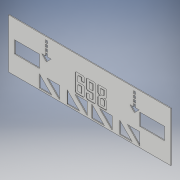
# Autodesk Inventor part: Lower Ramp
Saved by Autodesk Inventor 2018 (Build 220112000, 112)
## iProperties
Created: 2018-02-11
Part Number: Lower Ramp
Material: Generic
Document SubType Name: Modeling
Designer: Orangeracer
Density: 1 g/cm^3
Appearance: Default
Author: Orangeracer
Autodesk Inventor part; units mm, degrees
ref_plane "YZ Plane" through (0, 0, 0) normal (1, 0, 0) x (0, 1, 0)
ref_plane "XZ Plane" through (0, 0, 0) normal (0, 1, 0) x (-1, 0, 0)
ref_plane "XY Plane" through (0, 0, 0) normal (0, 0, 1) x (1, 0, 0)
sketch "Sketch1" plane through (0, 0, 0) normal (0, 0, 1) x (1, 0, 0)
  line L0 (0, 0) -> (666.75, 0)
  line L1 (666.75, 0) -> (666.75, -76.2)
  line L2 (666.75, -76.2) -> (0, -76.2)
  line L3 (0, -76.2) -> (0, 0)
  line L4 (127, 0) -> (539.75, 0)
  line L5 (539.75, 0) -> (539.75, 50.8)
  line L6 (539.75, 50.8) -> (127, 50.8)
  line L7 (127, 50.8) -> (127, 0)
  line L8 (0, 50.8) -> (666.75, 50.8)
  line L9 (666.75, 50.8) -> (666.75, 127)
  line L10 (666.75, 127) -> (0, 127)
  line L11 (0, 127) -> (0, 50.8)
  line L12 (25.4, 50.8) -> (0, 50.8)
  line L13 (0, 50.8) -> (0, 0)
  line L14 (0, 0) -> (25.4, 0)
  line L15 (25.4, 0) -> (25.4, 50.8)
  line L16 (666.75, 50.8) -> (641.35, 50.8)
  line L17 (641.35, 50.8) -> (641.35, 0)
  line L18 (641.35, 0) -> (666.75, 0)
  line L19 (666.75, 0) -> (666.75, 50.8)
  dimension "d0" = 666.75
  dimension "d1" = 76.2
  dimension "d2" = 50.8
  dimension "d3" = 666.75
  dimension "d4" = 0
  dimension "d5" = 76.2
  dimension "d6" = 127
  dimension "d7" = 127
  dimension "d8" = 25.4
  dimension "d9" = 50.8
  dimension "d10" = 25.4
  constraints: 40 end point, 10 parallel, 5 horizontal, 5 perpendicular, 4 point on line
  measures "d0" distance of L1.end L2.end
  measures "d1" distance of L0.end L1.end
  measures "d2" distance of L6.end L4.start
  measures "d3" distance of L9.end L10.end
  measures "d4" distance between parallel lines of L1 L9
  measures "d5" distance of L10.end L8.start
  measures "d6" distance between parallel lines of L3 L7
  measures "d7" distance between parallel lines of L9 L5
  measures "d8" distance between parallel lines of L13 L15
  measures "d9" distance of L12.end L0.start
  measures "d10" distance between parallel lines of L19 L17
extrude "Extrusion1" add sketch "Sketch1" along normal blind 3.175 contours L13 L8 L15 L0 | L0 L1 L2 L3 | L11 L10 L9 L8 L6 | L7 L6 L5 L0 | L0 L17 L8 L19
sketch "Sketch2" plane through (0, 0, 3.175) normal (0, 0, 1) x (1, 0, 0)
  line L0 (269.875, 63.5) -> (563.8865, 63.5) construction
  line L1 (563.8865, 63.5) -> (563.8865, -18.7489) construction
  line L2 (563.8865, -18.7489) -> (269.875, -18.7489) construction
  line L3 (269.875, -18.7489) -> (269.875, 63.5) construction
  line L4 (127, 50.8) -> (127, 0) projected
  line L5 (666.75, 127) -> (0, 127) projected
  spline S0 degree 2 poles (311.2942, -6.6857) (311.2942, -12.7) (305.2799, -12.7) knots 0 0 0 1 1 1
  line L6 (305.2799, -12.7) -> (280.4851, -12.7)
  spline S1 degree 2 poles (280.4851, -12.7) (274.4708, -12.7) (274.4708, -6.6857) knots 0 0 0 1 1 1
  line L7 (274.4708, -6.6857) -> (274.4708, 57.4857)
  spline S2 degree 2 poles (274.4708, 57.4857) (274.4708, 63.5) (280.3716, 63.5) knots 0 0 0 1 1 1
  line L8 (280.3716, 63.5) -> (305.053, 63.5)
  spline S3 degree 2 poles (305.053, 63.5) (311.124, 63.5) (311.124, 57.4857) knots 0 0 0 1 1 1
  line L9 (311.124, 57.4857) -> (311.124, 40.4074)
  line L10 (311.124, 40.4074) -> (299.9465, 40.4074)
  line L11 (299.9465, 40.4074) -> (299.9465, 53.741)
  line L12 (299.9465, 53.741) -> (285.6483, 53.741)
  line L13 (285.6483, 53.741) -> (285.6483, 30.8185)
  line L14 (285.6483, 30.8185) -> (305.2799, 30.8185)
  spline S4 degree 2 poles (305.2799, 30.8185) (311.2942, 30.8185) (311.2942, 24.8042) knots 0 0 0 1 1 1
  line L15 (311.2942, 24.8042) -> (311.2942, -6.6857)
  line L16 (300.1734, -2.941) -> (300.1734, 21.1162)
  line L17 (300.1734, 21.1162) -> (285.6483, 21.1162)
  line L18 (285.6483, 21.1162) -> (285.6483, -2.941)
  line L19 (285.6483, -2.941) -> (300.1734, -2.941)
  spline S5 degree 2 poles (357.139, -6.6857) (357.139, -12.7) (351.1247, -12.7) knots 0 0 0 1 1 1
  line L20 (351.1247, -12.7) -> (326.2165, -12.7)
  spline S6 degree 2 poles (326.2165, -12.7) (320.4859, -12.7) (320.4859, -6.6857) knots 0 0 0 1 1 1
  line L21 (320.4859, -6.6857) -> (320.4859, 10.3926)
  line L22 (320.4859, 10.3926) -> (331.6634, 10.3926)
  line L23 (331.6634, 10.3926) -> (331.6634, -2.941)
  line L24 (331.6634, -2.941) -> (345.848, -2.941)
  line L25 (345.848, -2.941) -> (345.848, 19.9815)
  line L26 (345.848, 19.9815) -> (325.8193, 19.9815)
  spline S7 degree 2 poles (325.8193, 19.9815) (320.2022, 19.9815) (320.2022, 25.9958) knots 0 0 0 1 1 1
  line L27 (320.2022, 25.9958) -> (320.2022, 57.4857)
  spline S8 degree 2 poles (320.2022, 57.4857) (320.2022, 63.5) (325.8193, 63.5) knots 0 0 0 1 1 1
  line L28 (325.8193, 63.5) -> (351.0113, 63.5)
  spline S9 degree 2 poles (351.0113, 63.5) (357.139, 63.5) (357.139, 57.4857) knots 0 0 0 1 1 1
  line L29 (357.139, 57.4857) -> (357.139, -6.6857)
  line L30 (345.848, 29.627) -> (345.848, 53.741)
  line L31 (345.848, 53.741) -> (331.323, 53.741)
  line L32 (331.323, 53.741) -> (331.323, 29.627)
  line L33 (331.323, 29.627) -> (345.848, 29.627)
  spline S10 degree 2 poles (403.9484, -6.6857) (403.9484, -12.7) (397.9341, -12.7) knots 0 0 0 1 1 1
  line L34 (397.9341, -12.7) -> (372.2883, -12.7)
  spline S11 degree 2 poles (372.2883, -12.7) (366.274, -12.7) (366.274, -6.6857) knots 0 0 0 1 1 1
  line L35 (366.274, -6.6857) -> (366.274, 16.4069)
  spline S12 degree 2 poles (366.274, 16.4069) (366.274, 20.6056) (369.1109, 22.8751) knots 0 0 0 1 1 1
  spline S13 degree 2 poles (369.1109, 22.8751) (372.4585, 24.8042) (375.8628, 26.7901) knots 0 0 0 1 1 1
  spline S14 degree 2 poles (375.8628, 26.7901) (372.5719, 28.6625) (369.3378, 30.5916) knots 0 0 0 1 1 1
  spline S15 degree 2 poles (369.3378, 30.5916) (366.3874, 32.9179) (366.3874, 36.8896) knots 0 0 0 1 1 1
  line L36 (366.3874, 36.8896) -> (366.3874, 57.4857)
  spline S16 degree 2 poles (366.3874, 57.4857) (366.3874, 63.5) (372.5719, 63.5) knots 0 0 0 1 1 1
  line L37 (372.5719, 63.5) -> (397.8206, 63.5)
  spline S17 degree 2 poles (397.8206, 63.5) (403.7782, 63.5) (403.7782, 57.4857) knots 0 0 0 1 1 1
  line L38 (403.7782, 57.4857) -> (403.7782, 36.8896)
  spline S18 degree 2 poles (403.7782, 36.8896) (403.7782, 32.8611) (400.8278, 30.5916) knots 0 0 0 1 1 1
  spline S19 degree 2 poles (400.8278, 30.5916) (397.5937, 28.6625) (394.3028, 26.7901) knots 0 0 0 1 1 1
  spline S20 degree 2 poles (394.3028, 26.7901) (397.6504, 24.8042) (401.0547, 22.8751) knots 0 0 0 1 1 1
  spline S21 degree 2 poles (401.0547, 22.8751) (403.9484, 20.6056) (403.9484, 16.4069) knots 0 0 0 1 1 1
  line L39 (403.9484, 16.4069) -> (403.9484, -6.6857)
  line L40 (392.6007, -3.1112) -> (392.6007, 17.9956)
  line L41 (392.6007, 17.9956) -> (385.1112, 22.3077)
  line L42 (385.1112, 22.3077) -> (377.5649, 17.9956)
  line L43 (377.5649, 17.9956) -> (377.5649, -3.1112)
  line L44 (377.5649, -3.1112) -> (392.6007, -3.1112)
  line L45 (392.4872, 35.6413) -> (392.4872, 53.9112)
  line L46 (392.4872, 53.9112) -> (377.7352, 53.9112)
  line L47 (377.7352, 53.9112) -> (377.7352, 35.6413)
  line L48 (377.7352, 35.6413) -> (385.1112, 31.2725)
  line L49 (385.1112, 31.2725) -> (392.4872, 35.6413)
  point P0 (0, 0)
  dimension "d26" = 142.875
  dimension "d27" = 63.5
  constraints: 2 other
  measures "d26" distance between parallel lines of L4 L3
  measures "d27" distance between parallel lines of L5 L0
extrude "Extrusion2" cut sketch "Sketch2" against normal blind 1.5748
sketch "Sketch3" plane through (0, 0, 3.175) normal (0, 0, 1) x (1, 0, 0)
  line L0 (127, -19.05) -> (127, -69.85)
  line L1 (127, -69.85) -> (177.8, -69.85)
  line L2 (177.8, -69.85) -> (127, -19.05)
  line L3 (0, -76.2) -> (666.75, -76.2) projected
  line L4 (127, 50.8) -> (127, 0) projected
  line L5 (158.75, -19.05) -> (209.55, -19.05)
  line L6 (209.55, -19.05) -> (209.55, -69.85)
  line L7 (209.55, -69.85) -> (158.75, -19.05)
  line L8 (241.3, -19.05) -> (241.3, -69.85)
  line L9 (241.3, -69.85) -> (292.1, -69.85)
  line L10 (292.1, -69.85) -> (241.3, -19.05)
  line L11 (273.05, -19.05) -> (323.85, -19.05)
  line L12 (323.85, -19.05) -> (323.85, -69.85)
  line L13 (323.85, -69.85) -> (273.05, -19.05)
  line L14 (342.9, -19.05) -> (342.9, -69.85)
  line L15 (342.9, -69.85) -> (393.7, -69.85)
  line L16 (374.65, -19.05) -> (425.45, -19.05)
  line L17 (425.45, -19.05) -> (425.45, -69.85)
  line L18 (425.45, -69.85) -> (374.65, -19.05)
  line L19 (393.7, -69.85) -> (342.9, -19.05)
  line L20 (457.2, -69.85) -> (457.2, -19.05)
  line L21 (457.2, -19.05) -> (508, -69.85)
  line L22 (508, -69.85) -> (457.2, -69.85)
  line L23 (488.95, -19.05) -> (539.75, -19.05)
  line L24 (539.75, -19.05) -> (539.75, -69.85)
  line L25 (539.75, -69.85) -> (488.95, -19.05)
  line L26 (539.75, 0) -> (539.75, 50.8) projected
  point P0 (0, 0)
  dimension "d36" = 50.8
  dimension "d37" = 50.8
  dimension "d38" = 71.8421
  dimension "d39" = 90
  dimension "d40" = 45
  dimension "d41" = 45
  dimension "d42" = 6.35
  dimension "d43" = 0
  dimension "d44" = 50.8
  dimension "d45" = 50.8
  dimension "d46" = 45
  dimension "d47" = 57.15
  dimension "d48" = 31.75
  dimension "d49" = 50.8
  dimension "d50" = 50.8
  dimension "d51" = 90
  dimension "d52" = 45
  dimension "d55" = 90
  dimension "d56" = 31.75
  dimension "d57" = 50.8
  dimension "d58" = 50.8
  dimension "d59" = 31.75
  dimension "d60" = 57.15
  dimension "d61" = 50.8
  dimension "d62" = 50.8
  dimension "d63" = 6.35
  dimension "d64" = 19.05
  dimension "d65" = 50.8
  dimension "d66" = 50.8
  dimension "d67" = 57.15
  dimension "d68" = 31.75
  dimension "d71" = 50.8
  dimension "d72" = 50.8
  dimension "d73" = 6.35
  dimension "d74" = 31.75
  dimension "d75" = 50.8
  dimension "d76" = 50.8
  dimension "d77" = 31.75
  dimension "d78" = 57.15
  dimension "d79" = 0
  constraints: 48 end point, 7 perpendicular, 4 horizontal, 3 vertical
  measures "d36" distance of L0.end L1.end
  measures "d37" distance of L0.start L0.end
  measures "d38" distance of L1.end L0.start
  measures "d39" angle of L1 L0
  measures "d40" angle of L1 L2
  measures "d41" angle of L2 L0
  measures "d42" distance between parallel lines of L3 L1
  measures "d43" distance between parallel lines of L4 L0
  measures "d44" distance of L5.start L5.end
  measures "d45" distance of L5.end L6.end
  measures "d46" angle of L6 L7
  measures "d47" distance between parallel lines of L3 L5
  measures "d48" distance of L1.end L6.end
  measures "d49" distance of L8.start L8.end
  measures "d50" distance of L8.end L9.end
  measures "d51" angle of L9 L8
  measures "d52" angle of L10 L8
  measures "d55" angle of L6 L5
  measures "d56" distance between parallel lines of L6 L8
  measures "d57" distance of L11.end L12.end
  measures "d58" distance of L11.start L11.end
  measures "d59" distance of L9.end L12.end
  measures "d60" distance between parallel lines of L3 L11
  measures "d61" distance of L14.start L14.end
  measures "d62" distance of L14.end L15.end
  measures "d63" distance between parallel lines of L3 L15
  measures "d64" distance between parallel lines of L12 L14
  measures "d65" distance of L16.end L17.end
  measures "d66" distance of L16.start L16.end
  measures "d67" distance between parallel lines of L3 L16
  measures "d68" distance of L15.end L17.end
  measures "d71" distance of L20.start L20.end
  measures "d72" distance of L21.end L20.start
  measures "d73" distance between parallel lines of L3 L22
  measures "d74" distance between parallel lines of L17 L20
  measures "d75" distance of L23.start L23.end
  measures "d76" distance of L23.end L24.end
  measures "d77" distance of L21.end L24.end
  measures "d78" distance between parallel lines of L3 L23
  measures "d79" distance between parallel lines of L26 L24
extrude "Extrusion3" cut sketch "Sketch3" against normal blind 25.4
sketch "Sketch4" plane through (0, 0, 3.175) normal (0, 0, 1) x (1, 0, 0)
  line L0 (488.95, 114.3) -> (539.75, 114.3) construction
  line L1 (539.75, 114.3) -> (539.75, 65.8025) construction
  line L2 (539.75, 65.8025) -> (488.95, 65.8025) construction
  line L3 (488.95, 65.8025) -> (488.95, 114.3) construction
  line L4 (127, 65.895) -> (127, 114.3) construction
  line L5 (127, 114.3) -> (177.8, 114.3) construction
  line L6 (177.8, 114.3) -> (177.8, 65.895) construction
  line L7 (177.8, 65.895) -> (127, 65.895) construction
  line L8 (127, 50.8) -> (127, 0) projected
  line L9 (539.75, 0) -> (539.75, 50.8) projected
  line L10 (666.75, 127) -> (0, 127) projected
  line L11 (156.1905, 38.1) -> (137.1405, 57.15)
  line L12 (137.1405, 57.15) -> (152.3805, 57.15)
  line L13 (152.3805, 57.15) -> (152.3805, 68.58)
  line L14 (152.3805, 68.58) -> (160.0005, 68.58)
  line L15 (160.0005, 68.58) -> (160.0005, 57.15)
  line L16 (160.0005, 57.15) -> (175.2405, 57.15)
  line L17 (175.2405, 57.15) -> (156.1905, 38.1)
  line L18 (152.3805, 88.9195) -> (152.3805, 99.06)
  line L19 (152.3805, 99.06) -> (160.0005, 99.06)
  line L20 (160.0005, 99.06) -> (160.0005, 88.9195)
  line L21 (160.0005, 88.9195) -> (152.3805, 88.9195)
  line L22 (152.3805, 73.6795) -> (152.3805, 83.82)
  line L23 (152.3805, 83.82) -> (160.0005, 83.82)
  line L24 (160.0005, 83.82) -> (160.0005, 73.6795)
  line L25 (160.0005, 73.6795) -> (152.3805, 73.6795)
  line L26 (152.3805, 104.1595) -> (152.3805, 114.3)
  line L27 (152.3805, 114.3) -> (160.0005, 114.3)
  line L28 (160.0005, 114.3) -> (160.0005, 104.1595)
  line L29 (160.0005, 104.1595) -> (152.3805, 104.1595)
  line L30 (518.1405, 38.1) -> (499.0905, 57.15)
  line L31 (499.0905, 57.15) -> (514.3305, 57.15)
  line L32 (514.3305, 57.15) -> (514.3305, 68.58)
  line L33 (514.3305, 68.58) -> (521.9505, 68.58)
  line L34 (521.9505, 68.58) -> (521.9505, 57.15)
  line L35 (521.9505, 57.15) -> (537.1905, 57.15)
  line L36 (537.1905, 57.15) -> (518.1405, 38.1)
  line L37 (514.3305, 104.1595) -> (514.3305, 114.3)
  line L38 (514.3305, 114.3) -> (521.9505, 114.3)
  line L39 (521.9505, 114.3) -> (521.9505, 104.1595)
  line L40 (521.9505, 104.1595) -> (514.3305, 104.1595)
  line L41 (514.3305, 73.6795) -> (514.3305, 83.82)
  line L42 (514.3305, 83.82) -> (521.9505, 83.82)
  line L43 (521.9505, 83.82) -> (521.9505, 73.6795)
  line L44 (521.9505, 73.6795) -> (514.3305, 73.6795)
  line L45 (514.3305, 88.9195) -> (514.3305, 99.06)
  line L46 (514.3305, 99.06) -> (521.9505, 99.06)
  line L47 (521.9505, 99.06) -> (521.9505, 88.9195)
  line L48 (521.9505, 88.9195) -> (514.3305, 88.9195)
  point P0 (0, 0)
  dimension "d82" = 0
  dimension "d83" = 50.8
  dimension "d84" = 50.8
  dimension "d85" = 0
  dimension "d86" = 12.7
  dimension "d87" = 12.7
  constraints: 4 other
  measures "d82" distance between parallel lines of L8 L4
  measures "d83" distance between parallel lines of L6 L4
  measures "d84" distance between parallel lines of L1 L3
  measures "d85" distance between parallel lines of L9 L1
  measures "d86" distance between parallel lines of L10 L0
  measures "d87" distance between parallel lines of L10 L5
extrude "Extrusion4" cut sketch "Sketch4" against normal blind 25.4
body "Solid1"
